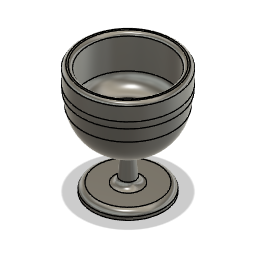
GB - Trofeo 3er puesto v8 (Autodesk Fusion 360 design; units mm, degrees)
Autodesk Fusion 360 part; units mm, degrees
note: some values were not read from the file. Chosen so that the rebuilt part matches the saved one: which face or edge a step refers to; the sign of a taper.
sketch "Sketch15" plane through (0, 0, 0) normal (0, 1, 0) x (1, 0, 0)
  circle A0 centre (0, 0) radius 9
  line L0 (-3.6373, -2.1) -> (3.6373, -2.1)
  line L1 (3.6373, -2.1) -> (0, 4.2)
  line L2 (0, 4.2) -> (-3.6373, -2.1)
  dimension "d130" = 18
  dimension "d173" = 2.1
  constraint coincident A0.centre origin
  constraint horizontal L0
  measures "d130" diameter of A0
  measures "d173" distance of A0.centre L2
extrude "Extrude11" add sketch "Sketch15" along normal blind 2 contours A0 | L0 L1 L2
fillet "Fillet7" radius 1.25 1 edges at (-9, 2, 0)
sketch "Sketch16" plane through (0, 2, 0) normal (0, 1, 0) x (-1, 0, 0)
  circle A0 centre (0, 0) radius 2
  circle A1 centre (0, 0) radius 7.75
  dimension "d133" = 4
  measures "d133" diameter of A0
extrude "Extrude12" add sketch "Sketch16" along normal blind 8 contours A0
draft "Draft1" angle 5 neutral plane through (0, 2, 0) pull (0, 1, 0) 1 faces at (-1.9975, 7.3333, -0.0997)
sketch "Sketch17" plane through (0, 10, 0) normal (0, 1, 0) x (-1, 0, 0)
  circle A0 centre (0, 0) radius 1.3001
  circle A1 centre (0, 0) radius 12
  dimension "d147" = 24
  constraint concentric A0 A1
  measures "d147" diameter of A1
extrude "Extrude13" add sketch "Sketch17" along normal blind 18 contours A0 | A1
fillet "Fillet6" radius 1.5 2 edges at (1.3001, 10, 0) (2, 2, 0)
chamfer "Chamfer1" distance 13 distance2 2 1 edges at (11.1879, 10, -4.3394) measured on face at (-11.9851, 22, -0.5982)
fillet "Fillet5" radius 10.75 2 edges at (10, 10, 0) (12, 23, 0)
sketch "Sketch18" plane through (0, 28, 0) normal (0, 1, 0) x (-1, 0, 0)
  circle A0 centre (0, 0) radius 12
  circle A1 centre (0, 0) radius 10
  dimension "d141" = 2
  constraint concentric A0 A1
  measures "d141" distance of A0 A1
extrude "Extrude14" cut sketch "Sketch18" against normal blind 12 contours A1
fillet "Fillet8" radius 3.5 1 edges at (10, 16, 0)
sketch "Sketch19" plane through (0, 0, 0) normal (0, 0, 1) x (1, 0, 0)
  arc A0 (9.9149, 15.7283) -> (12, 23.8221) centre (13.4715, 19.1275) ccw
  line L0 (12, 28) -> (12, 0)
  line L1 (12, 28) -> (-12, 28)
  point P0 (12, 23.8221)
  constraint vertical L0
  constraint coincident L0.start L1
  constraint coincident L0 L1.start
  constraint coincident P0 L0
  constraint coincident P0 A0.end
fillet "Fillet9" radius 0.8 2 edges at (10, 28, 0) (12, 28, 0)
named bodies: "Trofeo 3er puesto"
